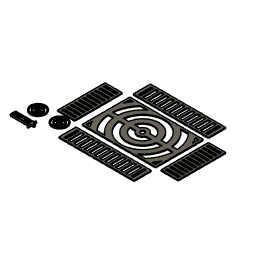
Bearhack Blood Bag Agitator Tray (Autodesk Fusion 360 design; units mm, degrees)
Autodesk Fusion 360 part; units mm, degrees
sketch "Sketch1" plane through (0, 0, 0) normal (0, 0, 1) x (1, 0, 0)
  line L0 (0, 0) -> (38, 0)
  line L1 (38, 0) -> (38, 8)
  line L2 (38, 8) -> (0, 8)
  line L3 (0, 8) -> (0, 0)
  circle A0 centre (19, 4) radius 4
  line L4 (19, 0) -> (38, 0)
  line L5 (-2, 10) -> (40, 10)
  line L6 (40, 10) -> (40, -2)
  line L7 (40, -2) -> (-2, -2)
  line L8 (-2, -2) -> (-2, 10)
  circle A1 centre (19, 4) radius 5
  constraint horizontal L0
  constraint vertical L1
  constraint horizontal L2
  constraint vertical L3
  constraint coincident L0.start L3.end
  constraint tangent L2 A0
  constraint midpoint L0 L4.start
  constraint tangent A0 L4
  constraint horizontal L5
  constraint vertical L6
  constraint horizontal L7
  constraint vertical L8
  constraint concentric A0 A1
extrude "Extrude1" add sketch "Sketch1" along normal blind 2 makes body 1
sketch "Sketch2" plane through (0, 0, 2) normal (0, 0, 1) x (-1, 0, 0)
  line L0 (-22, -8) -> (-38, -8)
  line L1 (-38, -8) -> (-38, 0)
  line L2 (-38, 0) -> (-22, 0)
  arc A0 (-16, 0) -> (-22, 0) centre (-19, -4) ccw
  line L3 (-16, 0) -> (0, 0)
  line L4 (0, 0) -> (0, -8)
  line L5 (0, -8) -> (-16, -8)
  arc A1 (-22, -8) -> (-16, -8) centre (-19, -4) ccw
  line L6 (2, 2) -> (-40, 2)
  line L7 (-40, 2) -> (-40, -10)
  line L8 (-40, -10) -> (2, -10)
  line L9 (2, -10) -> (2, 2)
  line L10 (2, -10) -> (-40, -10)
  line L11 (-40, -10) -> (-40, 2)
  line L12 (-40, 2) -> (2, 2)
  line L13 (2, 2) -> (2, -10)
  line L14 (0, -8) -> (-2, 0)
  line L15 (-3, -8) -> (-5, 0)
  line L16 (-8.5, -8) -> (-10.5, 0)
  line L17 (-5.5, -8) -> (-7.5, 0)
  line L18 (-14, -8) -> (-16, 0)
  line L19 (-11, -8) -> (-13, 0)
  line L20 (-38, 0) -> (-36, -8)
  line L21 (-35, 0) -> (-33, -8)
  line L22 (-32.5, 0) -> (-30.5, -8)
  line L23 (-29.5, 0) -> (-27.5, -8)
  line L24 (-27, 0) -> (-25, -8)
  line L25 (-24, 0) -> (-22, -8)
  circle A2 centre (-19, -4) radius 5
  dimension "d5" = -11
  dimension "d6" = 0
  dimension "d9" = 11
  dimension "d10" = 0
  constraint horizontal L10
  constraint vertical L11
  constraint horizontal L12
  constraint vertical L13
  constraint coincident L6.end L7.start
  constraint coincident L8.end L9.start
  constraint coincident L4.end L5.start
  constraint coincident L3 L14.end
  constraint coincident L5 L15.start
  constraint coincident L3 L15.end
  constraint coincident L1.end L2.start
  constraint coincident L0 L20.end
  constraint coincident L2 L21.start
  constraint coincident L0 L21.end
  constraint parallel L20 L21
  constraint concentric A0 A2
extrude "Extrude2" add sketch "Sketch2" along normal blind 2 contours L0 L2 L24 L25 A2 | L0 L2 L22 L23 | L3 L5 L18 L19 A2 | L0 L2 L20 L21 | L3 L5 L16 L17 | L3 L5 L14 L15 | L6 L7 L8 L9 L10 L11 L12 L13 bodies 1
extrude "Extrude3" add 1 faces at (40, 6, 1.3333) along direction (1, 0, 0) blind 3 on bodies 1 bodies 1
sketch "Sketch3" plane through (43, 0, 0) normal (1, 0, 0) x (0, 1, 0)
  line L0 (-2, 0) -> (10, 0)
  line L1 (10, 0) -> (10, 4)
  line L2 (10, 4) -> (-2, 4)
  line L3 (-2, 4) -> (-2, 0)
  line L4 (-2, 4) -> (10, 4)
  line L5 (10, 4) -> (10, 0)
  line L6 (10, 0) -> (-2, 0)
  line L7 (-2, 0) -> (-2, 4)
  line L8 (0, 4) -> (8, 4)
  line L9 (8, 4) -> (8, 0)
  line L10 (8, 0) -> (0, 0)
  line L11 (0, 0) -> (0, 4)
  constraint horizontal L4
  constraint vertical L5
  constraint horizontal L6
  constraint vertical L7
  constraint coincident L0.end L1.start
  constraint coincident L2.end L3.start
  constraint horizontal L8
  constraint vertical L9
  constraint horizontal L10
  constraint vertical L11
  constraint coincident L0 L9.end
  constraint coincident L2 L8.start
extrude "Extrude4" add sketch "Sketch3" along normal blind 3 contours L0 L2 L4 L6 L8 L9 L10 L11 bodies 1
sketch "Sketch4" plane through (0, -2, 0) normal (0, -1, 0) x (1, 0, 0)
  line L0 (-2, 0) -> (43, 0)
  line L1 (43, 0) -> (43, 4)
  line L2 (43, 4) -> (-2, 4)
  line L3 (-2, 4) -> (-2, 0)
  line L4 (43, 4) -> (41, 4)
  line L5 (41, 4) -> (41, 0)
  line L6 (41, 0) -> (43, 0)
  line L7 (43, 0) -> (43, 4)
  constraint horizontal L4
  constraint vertical L5
  constraint horizontal L6
  constraint vertical L7
  constraint coincident L0 L5.end
  constraint coincident L1.end L2.start
extrude "Extrude5" add sketch "Sketch4" along normal blind 4 contours L0 L1 L2 L4 L5 L6 L7 bodies 1
sketch "Sketch5" plane through (0, 10, 0) normal (0, 1, 0) x (-1, 0, 0)
  line L0 (-43, 0) -> (2, 0)
  line L1 (2, 0) -> (2, 4)
  line L2 (2, 4) -> (-43, 4)
  line L3 (-43, 4) -> (-43, 0)
  line L4 (-43, 4) -> (-41, 4)
  line L5 (-41, 4) -> (-41, 0)
  line L6 (-41, 0) -> (-43, 0)
  line L7 (-43, 0) -> (-43, 4)
  constraint horizontal L4
  constraint vertical L5
  constraint horizontal L6
  constraint vertical L7
  constraint coincident L0 L5.end
  constraint coincident L2.end L3.start
extrude "Extrude6" add sketch "Sketch5" along normal blind 4 contours L0 L2 L3 L4 L5 L6 L7 bodies 1
sketch "Sketch6" plane through (46, 0, 0) normal (1, 0, 0) x (0, 1, 0)
  line L0 (0, 0) -> (8, 0)
  line L1 (8, 0) -> (8, 4)
  line L2 (8, 4) -> (0, 4)
  line L3 (0, 4) -> (0, 0)
  line L4 (2, 4) -> (6, 4)
  line L5 (6, 4) -> (6, 0)
  line L6 (6, 0) -> (2, 0)
  line L7 (2, 0) -> (2, 4)
  constraint horizontal L4
  constraint vertical L5
  constraint horizontal L6
  constraint vertical L7
  constraint coincident L0 L5.end
  constraint coincident L2 L4.start
extrude "Extrude7" add sketch "Sketch6" along normal blind 2 contours L0 L2 L4 L5 L6 L7 bodies 1
sketch "Sketch7" plane through (48, 0, 0) normal (1, 0, 0) x (0, 1, 0)
  line L0 (2, 0) -> (6, 0)
  line L1 (6, 0) -> (6, 4)
  line L2 (6, 4) -> (2, 4)
  line L3 (2, 4) -> (2, 0)
  circle A0 centre (4, 2) radius 17
  line L4 (2, 4) -> (6, 4)
  line L5 (6, 4) -> (6, 0)
  line L6 (6, 0) -> (2, 0)
  line L7 (2, 0) -> (2, 4)
  constraint horizontal L4
  constraint vertical L5
  constraint horizontal L6
  constraint vertical L7
  constraint coincident L0.end L1.start
  constraint coincident L2.end L3.start
extrude "Extrude8" add sketch "Sketch7" against normal blind 2 separate body makes body 2
sketch "Sketch8" plane through (48, 0, 0) normal (1, 0, 0) x (0, 1, 0)
  line L0 (6, 0) -> (2, 0)
  line L1 (2, 0) -> (2, 4)
  line L2 (2, 4) -> (6, 4)
  line L3 (6, 4) -> (6, 0)
  circle A0 centre (4, 2) radius 17
  circle A1 centre (4, 2) radius 15
  line L4 (-12, 1) -> (20, 1)
  line L5 (20, 1) -> (20, 3)
  line L6 (20, 3) -> (-12, 3)
  line L7 (-12, 3) -> (-12, 1)
  line L8 (3, 18) -> (5, 18)
  line L9 (5, 18) -> (5, -14)
  line L10 (5, -14) -> (3, -14)
  line L11 (3, -14) -> (3, 18)
  circle A2 centre (4, 2) radius 11
  circle A3 centre (4, 2) radius 9
  circle A4 centre (4, 2) radius 5
  circle A5 centre (4, 2) radius 3
  constraint concentric A0 A1
  constraint horizontal L4
  constraint vertical L5
  constraint horizontal L6
  constraint vertical L7
  constraint horizontal L8
  constraint vertical L9
  constraint horizontal L10
  constraint vertical L11
  constraint concentric A0 A2
  constraint concentric A1 A3
  constraint concentric A3 A4
  constraint concentric A0 A5
extrude "Extrude9" cut sketch "Sketch8" against normal blind 3 contours L4 L9 A3 A4 | L4 L11 A3 A4 | L6 L9 A3 A4 | A1 L4 L9 A2 | A1 L4 L11 A2 | L6 L11 A3 A4 | A1 L6 L9 A2 | A1 L6 L11 A2 bodies 2
move_face "OffsetFaces1" offset -0.2 1 faces at (47.3333, 6, 1.3333) on bodies 2
move_face "OffsetFaces2" offset -0.2 1 faces at (47.3333, 3.4, 0) on bodies 2
move_face "OffsetFaces3" offset -0.2 1 faces at (47.3333, 2, 2.6) on bodies 2
move_face "OffsetFaces4" offset -0.2 1 faces at (47.3333, 4.7333, 4) on bodies 2
move_body "Move1" bodies 2 to x (0, 0, -1) y (0, 1, 0) z (1, 0, 0) at (17, 25, 48)
move_body "Move2" bodies 1 to x (1, 0, 0) y (0, -1, 0) z (0, 0, -1) at (0, -4, 3.6527)
move_body "Move3" bodies 1 to x (1, 0, 0) y (0, 1, 0) z (0, 0, 1) at (0, 0, 0.5)
move_body "Align1" bodies 1 to x (1, 0, 0) y (0, 1, 0) z (0, 0, 1) at (0, 0, -0.1527)
copy_body "CopyPasteBodies1" bodies 2 makes body 3
move_body "Move4" bodies 3 to x (1, 0, 0) y (0, 1, 0) z (0, 0, 1) at (50, 0, 0)
sketch "Sketch9" plane through (46, 0, 0) normal (1, 0, 0) x (0, 1, 0)
  line L0 (-10, 0) -> (-10, 4)
  line L1 (-10, 4) -> (-12, 4)
  line L2 (-12, 4) -> (-12, 0)
  line L3 (-12, 0) -> (-10, 0)
  line L4 (-12, 4) -> (-10, 4)
  line L5 (-10, 4) -> (-10, 0)
  line L6 (-10, 0) -> (-12, 0)
  line L7 (-12, 0) -> (-12, 4)
  line L8 (-6, 4) -> (-4, 4)
  line L9 (-4, 4) -> (-4, 0)
  line L10 (-4, 0) -> (-6, 0)
  line L11 (-6, 0) -> (-6, 4)
  constraint horizontal L4
  constraint vertical L5
  constraint horizontal L6
  constraint vertical L7
  constraint coincident L0.start L3.end
  constraint coincident L1.end L2.start
  constraint horizontal L8
  constraint vertical L9
  constraint horizontal L10
  constraint vertical L11
extrude "Extrude10" cut sketch "Sketch9" against normal blind 3 bodies 1
sketch "Sketch10" plane through (0, 0, 0) normal (0, 0, 1) x (1, 0, 0)
  line L0 (0, 0) -> (170, 0)
  line L1 (170, 0) -> (170, 110)
  line L2 (170, 110) -> (0, 110)
  line L3 (0, 110) -> (0, 0)
  line L4 (170, 0) -> (172, 0)
  line L5 (172, 0) -> (172, 110)
  line L6 (172, 110) -> (170, 110)
  line L7 (170, 110) -> (170, 0)
  line L8 (172, 110) -> (0, 110)
  line L9 (0, 110) -> (0, 112)
  line L10 (0, 112) -> (172, 112)
  line L11 (172, 112) -> (172, 110)
  line L12 (0, 112) -> (-2, 112)
  line L13 (-2, 112) -> (-2, 0)
  line L14 (-2, 0) -> (0, 0)
  line L15 (0, 0) -> (0, 112)
  line L16 (-2, 0) -> (172, 0)
  line L17 (172, 0) -> (172, -2)
  line L18 (172, -2) -> (-2, -2)
  line L19 (-2, -2) -> (-2, 0)
  constraint horizontal L0
  constraint vertical L1
  constraint horizontal L2
  constraint vertical L3
  constraint coincident L0.start L3.end
  constraint horizontal L4
  constraint vertical L5
  constraint horizontal L6
  constraint vertical L7
  constraint horizontal L8
  constraint vertical L9
  constraint horizontal L10
  constraint vertical L11
  constraint horizontal L12
  constraint vertical L13
  constraint horizontal L14
  constraint vertical L15
  constraint horizontal L16
  constraint vertical L17
  constraint horizontal L18
  constraint vertical L19
extrude "Extrude11" add sketch "Sketch10" along normal blind 40 separate body contours L3 L9 L12 L13 L14 L15 L16 | L0 L4 L14 L16 L17 L18 L19 | L1 L4 L5 L6 L7 L8 L16 | L2 L6 L8 L9 L10 L11 L15 makes body 4
sketch "Sketch11" plane through (0, 0, 0) normal (0, 0, 1) x (1, 0, 0)
  line L0 (0, 110) -> (170, 110)
  line L1 (170, 110) -> (170, 0)
  line L2 (170, 0) -> (0, 0)
  line L3 (0, 0) -> (0, 110)
  constraint horizontal L0
  constraint vertical L1
  constraint horizontal L2
  constraint vertical L3
extrude "Extrude12" add sketch "Sketch11" along normal blind 2 bodies 4
sketch "Sketch12" plane through (0, 0, 2) normal (0, 0, 1) x (-1, 0, 0)
  line L0 (0, 0) -> (-170, 0)
  line L1 (-170, 0) -> (-170, -110)
  line L2 (-170, -110) -> (0, -110)
  line L3 (0, -110) -> (0, 0)
  circle A0 centre (-85, -55) radius 85
  circle A1 centre (-85, -55) radius 5
  dimension "d37" = 10
  constraint concentric A0 A1
  measures "d37" diameter of A1
extrude "Extrude13" cut sketch "Sketch12" against normal blind 2 contours A1 bodies 4
split "Split1" by plane through (170, 110, 0) normal (0, -1, 0) bodies 4 makes body 5 at (144.6667, 54.3333, 0)
split "Split2" by plane through (0, 0, 0) normal (0, 1, 0) bodies 5 makes body 6 at (144.6667, 55, 0)
split "Split3" by plane through (0, 110, 0) normal (1, 0, 0) bodies 6 makes body 7 at (144.6667, 55, 0)
split "Split4" by plane through (170, 0, 0) normal (-1, 0, 0) bodies 7 makes body 8 at (143.3333, 55, 0)
sketch "Sketch13" plane through (0, 0, 2) normal (0, 0, 1) x (-1, 0, 0)
  circle A0 centre (-85, -55) radius 5
  line L0 (0, 0) -> (-170, 0)
  line L1 (-170, 0) -> (-170, -110)
  line L2 (-170, -110) -> (0, -110)
  line L3 (0, -110) -> (0, 0)
  circle A1 centre (-85, -55) radius 25
  circle A2 centre (-85, -55) radius 12.5
  circle A3 centre (-85, -55) radius 37.5
  circle A4 centre (-85, -55) radius 50
  circle A5 centre (-85, -55) radius 62.5
  circle A6 centre (-85, -55) radius 75
  circle A7 centre (-85, -55) radius 87.5
  line L4 (0, -60) -> (-170, -60)
  line L5 (-170, -60) -> (-170, -50)
  line L6 (-170, -50) -> (0, -50)
  line L7 (0, -50) -> (0, -60)
  line L8 (0, -110) -> (-170, -110)
  line L9 (-170, -110) -> (-170, -105)
  line L10 (-170, -105) -> (0, -105)
  line L11 (0, -105) -> (0, -110)
  line L12 (0, -110) -> (-5, -110)
  line L13 (-5, -110) -> (-5, 0)
  line L14 (-5, 0) -> (0, 0)
  line L15 (0, 0) -> (0, -110)
  line L16 (-170, -110) -> (-165, -110)
  line L17 (-165, -110) -> (-165, 0)
  line L18 (-165, 0) -> (-170, 0)
  line L19 (-170, 0) -> (-170, -110)
  line L20 (0, 0) -> (-170, 0)
  line L21 (-170, 0) -> (-170, -5)
  line L22 (-170, -5) -> (0, -5)
  line L23 (0, -5) -> (0, 0)
  dimension "d40" = 50
  dimension "d41" = 25
  dimension "d42" = 75
  dimension "d43" = 100
  dimension "d44" = 125
  dimension "d45" = 150
  dimension "d46" = 175
  constraint concentric A0 A1
  constraint concentric A0 A2
  constraint concentric A1 A3
  constraint concentric A1 A4
  constraint concentric A4 A5
  constraint concentric A1 A6
  constraint concentric A4 A7
  constraint horizontal L4
  constraint vertical L5
  constraint horizontal L6
  constraint vertical L7
  constraint coincident L1 L5.end
  constraint horizontal L8
  constraint vertical L9
  constraint horizontal L10
  constraint vertical L11
  constraint coincident L1 L9.end
  constraint coincident L2.end L3.start
  constraint horizontal L12
  constraint vertical L13
  constraint horizontal L14
  constraint vertical L15
  constraint coincident L0 L13.end
  constraint horizontal L16
  constraint vertical L17
  constraint horizontal L18
  constraint vertical L19
  constraint coincident L0 L17.end
  constraint coincident L1.end L2.start
  constraint horizontal L20
  constraint vertical L21
  constraint horizontal L22
  constraint vertical L23
  constraint coincident L0.start L3.end
  measures "d40" diameter of A1
  measures "d41" diameter of A2
  measures "d42" diameter of A3
  measures "d43" diameter of A4
  measures "d44" diameter of A5
  measures "d45" diameter of A6
  measures "d46" diameter of A7
extrude "Extrude14" cut sketch "Sketch13" against normal blind 2 contours A1 A2 L6 | A1 A2 L4 | A3 A4 L6 | A3 A4 L4 | A5 A6 L6 L22 | A5 A6 L6 L22 | A5 A6 L4 L10 | A5 A6 L4 L10 | A7 L17 L22 | A7 L13 L22 | A7 L10 L17 | A7 L10 L13 bodies 8
sketch "Sketch14" plane through (0, -2, 0) normal (0, -1, 0) x (1, 0, 0)
  line L0 (-2, 0) -> (172, 0)
  line L1 (172, 0) -> (172, 40)
  line L2 (172, 40) -> (-2, 40)
  line L3 (-2, 40) -> (-2, 0)
  line L4 (-2, 40) -> (175, 40)
  line L5 (175, 40) -> (175, 35)
  line L6 (175, 35) -> (-2, 35)
  line L7 (-2, 35) -> (-2, 40)
  line L8 (-2, 0) -> (175, 0)
  line L9 (175, 0) -> (175, 5)
  line L10 (175, 5) -> (-2, 5)
  line L11 (-2, 5) -> (-2, 0)
  line L12 (-2, 40) -> (5, 40)
  line L13 (5, 40) -> (5, -5)
  line L14 (5, -5) -> (-2, -5)
  line L15 (-2, -5) -> (-2, 40)
  line L16 (172, 40) -> (165, 40)
  line L17 (165, 40) -> (165, -5)
  line L18 (165, -5) -> (172, -5)
  line L19 (172, -5) -> (172, 40)
  line L20 (10, 35) -> (15, 35)
  line L21 (15, 35) -> (15, 5)
  line L22 (15, 5) -> (10, 5)
  line L23 (10, 5) -> (10, 35)
  line L24 (22.0833, 5) -> (22.0833, 35)
  line L25 (27.0833, 35) -> (27.0833, 5)
  line L26 (34.1667, 5) -> (34.1667, 35)
  line L27 (39.1667, 35) -> (39.1667, 5)
  line L28 (46.25, 5) -> (46.25, 35)
  line L29 (51.25, 35) -> (51.25, 5)
  line L30 (58.3333, 5) -> (58.3333, 35)
  line L31 (63.3333, 35) -> (63.3333, 5)
  line L32 (70.4167, 5) -> (70.4167, 35)
  line L33 (75.4167, 35) -> (75.4167, 5)
  line L34 (82.5, 5) -> (82.5, 35)
  line L35 (87.5, 35) -> (87.5, 5)
  line L36 (94.5833, 5) -> (94.5833, 35)
  line L37 (99.5833, 35) -> (99.5833, 5)
  line L38 (106.6667, 5) -> (106.6667, 35)
  line L39 (111.6667, 35) -> (111.6667, 5)
  line L40 (118.75, 5) -> (118.75, 35)
  line L41 (123.75, 35) -> (123.75, 5)
  line L42 (130.8333, 5) -> (130.8333, 35)
  line L43 (135.8333, 35) -> (135.8333, 5)
  line L44 (142.9167, 5) -> (142.9167, 35)
  line L45 (147.9167, 35) -> (147.9167, 5)
  line L46 (155, 5) -> (155, 35)
  line L47 (160, 35) -> (160, 5)
  dimension "d51" = 145
  dimension "d52" = 0
  constraint horizontal L4
  constraint vertical L5
  constraint horizontal L6
  constraint vertical L7
  constraint coincident L2.end L3.start
  constraint horizontal L8
  constraint vertical L9
  constraint horizontal L10
  constraint vertical L11
  constraint coincident L0.start L3.end
  constraint horizontal L12
  constraint vertical L13
  constraint horizontal L14
  constraint vertical L15
  constraint horizontal L16
  constraint vertical L17
  constraint horizontal L18
  constraint vertical L19
  constraint coincident L1.end L2.start
  constraint horizontal L20
  constraint vertical L21
  constraint horizontal L22
  constraint vertical L23
  constraint coincident L10 L21.end
  constraint coincident L6 L20.start
extrude "Extrude15" cut sketch "Sketch14" against normal blind 200 contours L6 L10 L13 L23 | L6 L10 L17 L47 | L6 L10 L21 L24 | L6 L10 L45 L46 | L6 L10 L25 L26 | L6 L10 L43 L44 | L6 L10 L27 L28 | L6 L10 L41 L42 | L6 L10 L29 L30 | L6 L10 L39 L40 | L6 L10 L31 L32 | L6 L10 L37 L38 | L6 L10 L33 L34 | L6 L10 L35 L36 bodies 4 5
sketch "Sketch15" plane through (172, 0, 0) normal (1, 0, 0) x (0, 1, 0)
  line L0 (0, 40) -> (0, 0)
  line L1 (0, 0) -> (110, 0)
  line L2 (110, 0) -> (110, 40)
  line L3 (110, 40) -> (0, 40)
  line L4 (0, 40) -> (5, 40)
  line L5 (5, 40) -> (5, 0)
  line L6 (5, 0) -> (0, 0)
  line L7 (0, 0) -> (0, 40)
  line L8 (0, 40) -> (110, 40)
  line L9 (110, 40) -> (110, 35)
  line L10 (110, 35) -> (0, 35)
  line L11 (0, 35) -> (0, 40)
  line L12 (110, 40) -> (105, 40)
  line L13 (105, 40) -> (105, 0)
  line L14 (105, 0) -> (110, 0)
  line L15 (110, 0) -> (110, 40)
  line L16 (110, 0) -> (0, 0)
  line L17 (0, 0) -> (0, 5)
  line L18 (0, 5) -> (110, 5)
  line L19 (110, 5) -> (110, 0)
  line L20 (10, 35) -> (15, 35)
  line L21 (15, 35) -> (15, 5)
  line L22 (15, 5) -> (10, 5)
  line L23 (10, 5) -> (10, 35)
  line L24 (24.4444, 35) -> (24.4444, 5)
  line L25 (19.4444, 5) -> (19.4444, 35)
  line L26 (33.8889, 35) -> (33.8889, 5)
  line L27 (28.8889, 5) -> (28.8889, 35)
  line L28 (43.3333, 35) -> (43.3333, 5)
  line L29 (38.3333, 5) -> (38.3333, 35)
  line L30 (52.7778, 35) -> (52.7778, 5)
  line L31 (47.7778, 5) -> (47.7778, 35)
  line L32 (62.2222, 35) -> (62.2222, 5)
  line L33 (57.2222, 5) -> (57.2222, 35)
  line L34 (71.6667, 35) -> (71.6667, 5)
  line L35 (66.6667, 5) -> (66.6667, 35)
  line L36 (81.1111, 35) -> (81.1111, 5)
  line L37 (76.1111, 5) -> (76.1111, 35)
  line L38 (90.5556, 35) -> (90.5556, 5)
  line L39 (85.5556, 5) -> (85.5556, 35)
  line L40 (100, 35) -> (100, 5)
  line L41 (95, 5) -> (95, 35)
  dimension "d57" = 85
  dimension "d58" = 85
  constraint horizontal L4
  constraint vertical L5
  constraint horizontal L6
  constraint vertical L7
  constraint coincident L1 L5.end
  constraint coincident L0.start L3.end
  constraint horizontal L8
  constraint vertical L9
  constraint horizontal L10
  constraint vertical L11
  constraint coincident L2 L9.end
  constraint horizontal L12
  constraint vertical L13
  constraint horizontal L14
  constraint vertical L15
  constraint coincident L1 L13.end
  constraint coincident L2.end L3.start
  constraint horizontal L16
  constraint vertical L17
  constraint horizontal L18
  constraint vertical L19
  constraint coincident L7 L17.end
  constraint coincident L1.end L2.start
  constraint horizontal L20
  constraint vertical L21
  constraint horizontal L22
  constraint vertical L23
  constraint coincident L18 L21.end
  constraint coincident L10 L20.start
extrude "Extrude16" cut sketch "Sketch15" against normal blind 200 contours L5 L10 L18 L23 | L10 L13 L18 L40 | L10 L18 L21 L25 | L10 L18 L38 L41 | L10 L18 L24 L27 | L10 L18 L36 L39 | L10 L18 L26 L29 | L10 L18 L34 L37 | L10 L18 L28 L31 | L10 L18 L32 L35 | L10 L18 L30 L33 bodies 6 7
move_body "Move5" bodies 5 to x (1, 0, 0) y (0, 0, -1) z (0, 1, 0) at (0, -42, 38)
move_body "Move6" bodies 6 to x (0, 0, -1) y (0, 1, 0) z (1, 0, 0) at (-37, 0, 33)
move_body "Move7" bodies 7 to x (0, 0, 1) y (0, 1, 0) z (-1, 0, 0) at (212, 0, -132)
move_body "Move8" bodies 4 to x (1, 0, 0) y (0, 0, 1) z (0, -1, 0) at (0, 150, -70)
move_body "Align2" bodies 7 to x (1, 0, 0) y (0, 1, 0) z (0, 0, 1) at (0, 0, -38)
move_body "Align3" bodies 4 to x (1, 0, 0) y (0, 1, 0) z (0, 0, 1) at (0, 0, -40)
move_body "Align4" bodies 6 to x (1, 0, 0) y (0, 1, 0) z (0, 0, 1) at (0, 0, -33)
move_body "Align5" bodies 5 to x (1, 0, 0) y (0, 1, 0) z (0, 0, 1) at (0, 0, -38)
move_body "Move9" bodies 5 to x (1, 0, 0) y (0, 1, 0) z (0, 0, 1) at (0, -10, 0)
move_body "Move10" bodies 6 to x (1, 0, 0) y (0, 1, 0) z (0, 0, 1) at (-20, 0, 0)
move_body "Move11" bodies 4 to x (1, 0, 0) y (0, 1, 0) z (0, 0, 1) at (0, 10, 0)
move_body "Move12" bodies 7 to x (1, 0, 0) y (0, 1, 0) z (0, 0, 1) at (10, 0, 0)
move_body "Move13" bodies 3 2 1 to x (1, 0, 0) y (0, 1, 0) z (0, 0, 1) at (-100, -50, 0)
named bodies: "adapter", "holder", "holder (1)"
